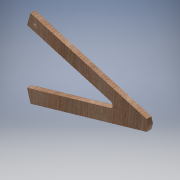
# Autodesk Inventor part: aFrameBase
Saved by Autodesk Inventor 2017 (Build 210142000, 142)
## iProperties
Created: 2017-04-28
Part Number: aFrameBase
Material: Generic
Document SubType Name: Modeling
Designer: admin
Density: 1 g/cm^3
Appearance: Birch - Natural Polished
Author: admin
Autodesk Inventor part; units mm, degrees
ref_plane "YZ Plane" through (0, 0, 0) normal (1, 0, 0) x (0, 1, 0)
ref_plane "XZ Plane" through (0, 0, 0) normal (0, 1, 0) x (-1, 0, 0)
ref_plane "XY Plane" through (0, 0, 0) normal (0, 0, 1) x (1, 0, 0)
ref_plane "Work Plane1" through (0, 0, 0) normal (0, 0, 1) x (1, 0, 0)
sketch "Sketch1" plane through (0, 0, 0) normal (0, 0, 1) x (1, 0, 0)
  line L0 (73.4542, 120.707) -> (75.2544, 119.6677) projected
  arc A0 (73.4542, 120.707) -> (70.7046, 122.2945) centre (72.0794, 121.5007) ccw projected
  line L1 (68.9044, 123.3338) -> (70.7046, 122.2945) projected
  line L2 (68.9044, 125.4125) -> (68.9044, 123.3338) projected
  arc A1 (68.9044, 125.4125) -> (68.9044, 128.5875) centre (68.9044, 127) ccw projected
  line L3 (68.9044, 130.6662) -> (68.9044, 128.5875) projected
  line L4 (70.7046, 131.7055) -> (68.9044, 130.6662) projected
  arc A2 (70.7046, 131.7055) -> (73.4542, 133.293) centre (72.0794, 132.4993) ccw projected
  line L5 (75.2544, 134.3323) -> (73.4542, 133.293) projected
  line L6 (77.0546, 133.293) -> (75.2544, 134.3323) projected
  arc A3 (77.0546, 133.293) -> (79.8042, 131.7055) centre (78.4294, 132.4993) ccw projected
  line L7 (81.6044, 130.6662) -> (79.8042, 131.7055) projected
  line L8 (81.6044, 128.5875) -> (81.6044, 130.6662) projected
  arc A4 (81.6044, 128.5875) -> (81.6044, 125.4125) centre (81.6044, 127) ccw projected
  line L9 (81.6044, 123.3338) -> (81.6044, 125.4125) projected
  line L10 (79.8042, 122.2945) -> (81.6044, 123.3338) projected
  arc A5 (79.8042, 122.2945) -> (77.0546, 120.707) centre (78.4294, 121.5007) ccw projected
  line L11 (75.2544, 119.6677) -> (77.0546, 120.707) projected
  circle A6 centre (75.2544, 127) radius 2.9337 projected
  line L12 (73.4542, -133.293) -> (75.2544, -134.3323) projected
  arc A7 (73.4542, -133.293) -> (70.7046, -131.7055) centre (72.0794, -132.4993) ccw projected
  line L13 (68.9044, -130.6662) -> (70.7046, -131.7055) projected
  line L14 (68.9044, -128.5875) -> (68.9044, -130.6662) projected
  arc A8 (68.9044, -128.5875) -> (68.9044, -125.4125) centre (68.9044, -127) ccw projected
  line L15 (68.9044, -123.3338) -> (68.9044, -125.4125) projected
  line L16 (70.7046, -122.2945) -> (68.9044, -123.3338) projected
  arc A9 (70.7046, -122.2945) -> (73.4542, -120.707) centre (72.0794, -121.5007) ccw projected
  line L17 (75.2544, -119.6677) -> (73.4542, -120.707) projected
  line L18 (77.0546, -120.707) -> (75.2544, -119.6677) projected
  arc A10 (77.0546, -120.707) -> (79.8042, -122.2945) centre (78.4294, -121.5007) ccw projected
  line L19 (81.6044, -123.3338) -> (79.8042, -122.2945) projected
  line L20 (81.6044, -125.4125) -> (81.6044, -123.3338) projected
  arc A11 (81.6044, -125.4125) -> (81.6044, -128.5875) centre (81.6044, -127) ccw projected
  line L21 (81.6044, -130.6662) -> (81.6044, -128.5875) projected
  line L22 (79.8042, -131.7055) -> (81.6044, -130.6662) projected
  arc A12 (79.8042, -131.7055) -> (77.0546, -133.293) centre (78.4294, -132.4993) ccw projected
  line L23 (75.2544, -134.3323) -> (77.0546, -133.293) projected
  circle A13 centre (75.2544, -127) radius 2.9337 projected
  line L24 (75.2544, -127) -> (513.2774, 0) construction
  line L25 (106.8774, 406.4) -> (106.8774, -406.4) projected
  line L26 (106.8774, 0) -> (513.2774, 0)
  line L27 (513.2774, 0) -> (75.2544, 127) construction
  line L28 (75.2544, 127) -> (68.1812, 102.6047) construction
  line L29 (75.2544, 127) -> (82.3275, 151.3953) construction
  line L30 (75.2544, 127) -> (50.8591, 134.0732) construction
  line L31 (82.3275, 151.3953) -> (57.9322, 158.4684)
  line L32 (57.9322, 158.4684) -> (50.8591, 134.0732)
  line L33 (50.8591, 134.0732) -> (43.7859, 109.6779)
  line L34 (43.7859, 109.6779) -> (68.1812, 102.6047)
  line L35 (82.3275, 151.3953) -> (513.2774, 26.4461)
  line L36 (68.1812, 102.6047) -> (164.7505, 74.6055)
  line L37 (538.647, 19.0904) -> (533.1119, 0)
  line L38 (524.5007, 29.7002) -> (513.2774, 26.4461)
  line L39 (43.7859, -109.6779) -> (57.9322, -158.4684)
  line L40 (57.9322, -158.4684) -> (513.2774, -26.4461)
  line L41 (538.647, -19.0904) -> (533.1119, 0)
  line L42 (266.3505, 45.1477) -> (379.9952, 12.1976)
  line L43 (164.7505, 74.6055) -> (266.3505, 45.1477)
  line L44 (164.7505, -74.6055) -> (43.7859, -109.6779)
  line L45 (266.3505, -45.1477) -> (164.7505, -74.6055)
  line L46 (379.9952, -12.1976) -> (266.3505, -45.1477)
  line L47 (379.9952, 12.1976) -> (513.2774, -26.4461) construction
  line L48 (513.2774, -26.4461) -> (524.5007, -29.7002)
  line L49 (513.2774, 26.4461) -> (526.5609, 22.5947)
  line L50 (513.2774, 26.4461) -> (379.9952, -12.1976) construction
  line L51 (513.2774, -26.4461) -> (538.647, -19.0904)
  arc A14 (379.9952, -12.1976) -> (379.9952, 12.1976) centre (376.4586, 0) ccw
  line L52 (526.5609, -22.5947) -> (524.5007, -29.7002)
  line L53 (526.5609, 22.5947) -> (538.647, 19.0904)
  line L54 (533.1119, 0) -> (526.5609, -22.5947)
  line L55 (533.1119, 0) -> (524.5007, 29.7002)
  point P0 (0, 0)
  dimension "d0" = 406.4
  dimension "d1" = 25.4
  dimension "d2" = 25.4
  dimension "d3" = 25.4
  dimension "d4" = 19.05
  dimension "d7" = 25.4
  dimension "d8" = 25.4
  dimension "d9" = 25.4
  dimension "d10" = 19.05
  dimension "d15" = 12.7
  constraints: 62 end point, 25 perpendicular, 15 parallel, 4 collinear, 4 point on line, 2 point on circle, 2 tangent, 1 centre point, 1 horizontal, 1 midpoint
  measures "d0" distance of L26.start L24.end
  measures "d1" distance of L27.end L28.end
  measures "d2" distance of L27.end L29.end
  measures "d3" distance of L27.end L30.end
  measures "d4" distance from line of L37 L24.end
  measures "d7" distance from line of L24.start L39
  measures "d8" distance from line of L40 L24.start
  measures "d9" distance from line of L38 L24.start
  measures "d10" distance from line of L24.end L41
  measures "d15" radius of A14
extrude "Extrusion1" add sketch "Sketch1" along normal blind 19.05 contours A7 L13 L14 A8 L15 L16 A9 L17 L18 A10 L19 L20 A11 L21 L22 A12 L23 L12 | A13 | L35 L49 L55 L54 L51 L40 L25 L44 L45 L46 A14 L42 L43 L36 | L25 L36 L34 L33 L32 L31 L35 | L25 L40 L39 L44
body "Solid1"
